3.2mm_funnel (Autodesk Fusion 360 design; units mm, degrees)
Autodesk Fusion 360 part; units mm, degrees
sketch "Sketch1" plane through (0, 0, 0) normal (0, 1, 0) x (1, 0, 0)
  line L0 (0, -1.8) -> (0, -10)
  line L1 (0, -10) -> (-22.5, -10)
  line L2 (-22.5, -10) -> (-22.5, -8)
  line L3 (-22.5, -8) -> (-17, -1.35)
  line L4 (-17, -1.35) -> (-16, -1.35)
  line L5 (-16, -1.35) -> (-16, -1.8)
  line L6 (-16, -1.8) -> (0, -1.8)
  dimension "d1" = 22.5
  dimension "d2" = 10
  dimension "d5" = 2
  dimension "d7" = 1.35
  dimension "d8" = 1.8
  dimension "d9" = 1
  dimension "d10" = 16
  constraint vertical L0
  constraint perpendicular L0 L1
  constraint perpendicular L1 L2
  constraint coincident origin L0
  constraint horizontal L4
  constraint perpendicular L4 L5
  constraint horizontal L6
  measures "d1" distance of L0.end L1.end
  measures "d2" distance of origin L1
  measures "d5" distance of L1.end L2.end
  measures "d7" vertical distance of origin L3.end
  measures "d8" distance of origin L6
  measures "d9" distance of L3.end L4.end
  measures "d10" distance of L0.start L5.end
revolve "Revolve1" add sketch "Sketch1" angle 360 about axis through (1.75, 0, 0) along (1, 0, 0)
chamfer "Chamfer1" distance 2 angle 45 1 edges at (0, -0.6509, -1.6782)
sketch "Sketch3" plane through (0, 0, 0) normal (1, 0, 0) x (0, 1, 0)
  circle A0 centre (0, 0) radius 10
  circle A1 centre (0, 0) radius 3.8
  line L0 (-5.5, 2.6875) -> (5.5, 2.6875) construction
  line L1 (5.5, 2.6875) -> (5.5, 7.0551) construction
  line L2 (5.5, 7.0551) -> (-5.5, 7.0551) construction
  line L3 (-5.5, 7.0551) -> (-5.5, 2.6875) construction
  point P0 (0, 7.0551)
  dimension "d15" = 2.2
  text T0 "3.2 mm" font "Arial" height 2.2 align centre top in box 11 x 4.3676 at (-5.5, 2.6875) x (1, 0) y (0, 1) spacing 1
  constraint midpoint L2 P0
  constraint vertical A0.centre
  constraint vertical P0
emboss "Emboss1" depth -0.4 profiles "Sketch3" section 1 text T0 onto face at (0, 0.4968, 7.8961)
sketch "Sketch4" plane through (0, 0, 0) normal (0, 1, 0) x (1, 0, 0)
  line L0 (-18.0003, 3.0001) -> (-4.0007, 3.0016) construction
  line L1 (-4.0007, 3.0016) -> (-4, -2.9986) construction
  line L2 (-4, -2.9986) -> (-17.9997, -3.0001) construction
  line L3 (-17.9997, -3.0001) -> (-18.0003, 3.0001) construction
  dimension "d20" = 2.5
  text T0 "3.2 mm" font "Arial" height 2.5 align centre middle in box 13.9996 x 6.0002 at (-18.0003, 3.0001) x (1, 0.000108) y (0.000108, -1) spacing 1 mirrored across
emboss "Emboss2" depth 0.2 profiles "Sketch4" section 1 text T0 onto face at (-15, 0.9957, 9.9503)
pattern_circular "C-Pattern1" count 3 over 360 about axis through (1.75, 0, 0) along (1, 0, 0) of "Emboss2"
fillet "Fillet1" radius 0.5 2 edges at (0, -3.6162, -9.3233) (-22.5, -3.6162, -9.3233)
equation "d7 = ( 2.7 / 2 ) * 1 mm"
equation "d8 = ( 3.6 / 2 ) * 1 mm"
equation "d10 = 22.5 mm - 6.5 mm"
